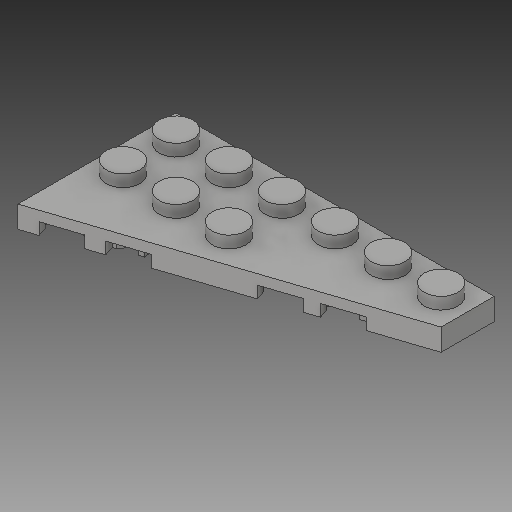
# Autodesk Inventor part: Grey triangle lego part
Saved by Autodesk Inventor 2017 (Build 210142000, 142)
## iProperties
Created: 2018-05-10
Part Number: Grey triangle lego part
Material: ABS Plastic
Document SubType Name: Modeling
Designer: 19000369
Density: 1.06 g/cm^3
Appearance: Light Gray
Mass: 1.84492 g
Surface Area: 27.5873 cm^2
Volume: 1.74049 cm^3
Author: 19000369
Autodesk Inventor part; units mm, degrees
ref_plane "YZ Plane" through (0, 0, 0) normal (1, 0, 0) x (0, 1, 0)
ref_plane "XZ Plane" through (0, 0, 0) normal (0, 1, 0) x (-1, 0, 0)
ref_plane "XY Plane" through (0, 0, 0) normal (0, 0, 1) x (1, 0, 0)
sketch "Sketch1" plane through (0, 0, 0) normal (0, 1, 0) x (-1, 0, 0)
  line L0 (0, 0) -> (0, -7.8486)
  line L1 (0, -7.8486) -> (47.0611, -7.8486)
  line L2 (47.0611, -7.8486) -> (47.0611, 15.5448)
  line L3 (47.0611, 15.5448) -> (0, 0)
  dimension "d0" = 7.8486
  dimension "d1" = 47.0611
  dimension "d2" = 23.3934
  constraints: 8 end point, 2 perpendicular, 1 vertical
  measures "d0" distance of L0.start L0.end
  measures "d1" distance of L0.end L1.end
  measures "d2" distance of L1.end L2.end
extrude "Extrusion1" add sketch "Sketch1" along normal blind 3.236
sketch "Sketch2" plane through (0, 3.236, 0) normal (0, 1, 0) x (1, 0, 0)
  circle A0 centre (-43.1394, 3.9268) radius 2.4867
  line L0 (-47.0611, 7.8486) -> (-47.0611, -15.5448) projected
  line L1 (0, 7.8486) -> (-47.0611, 7.8486) projected
  circle A1 centre (-43.1394, -3.9167) radius 2.4867
  circle A2 centre (-35.2958, 3.9268) radius 2.4867
  circle A3 centre (-35.2958, -3.9167) radius 2.4867
  circle A4 centre (-27.4523, 3.9268) radius 2.4867
  circle A5 centre (-27.4523, -3.9167) radius 2.4867
  circle A6 centre (-19.6088, 3.9268) radius 2.4867
  circle A7 centre (-19.6088, -3.9167) radius 2.4867
  circle A8 centre (-11.7653, 3.9268) radius 2.4867
  circle A9 centre (-11.7653, -3.9167) radius 2.4867
  circle A10 centre (-3.9218, 3.9268) radius 2.4867
  circle A11 centre (-3.9218, -3.9167) radius 2.4867
  dimension "d6" = 3.9218
  dimension "d7" = 3.9218
  dimension "d10" = 7.8435
  dimension "d13" = 7.8435
  constraints: 12 centre point, 1 horizontal, 1 vertical, 22 other
  measures "d6" distance from line of L0 A0.centre
  measures "d7" distance from line of L1 A0.centre
  measures "d10" distance of A0.centre A1.centre
  measures "d13" distance of A0.centre A2.centre
extrude "Extrusion2" add sketch "Sketch2" along normal blind 1.7577 contours A0 | A1 | A2 | A3 | A4 | A5 | A6 | A8 | A10
shell "Shell1" thickness 1.4732 removed faces 1 at (-31.3741, 0, 2.5654)
sketch "Sketch3" plane through (-45.5879, 1.7628, -6.3754) normal (0, -1, 0) x (1, 0, 0)
  circle A0 centre (5.8482, 6.3754) radius 2.4879
  circle A1 centre (13.8227, 6.3754) radius 2.4879
  circle A2 centre (21.5603, 6.3754) radius 2.4879
  circle A3 centre (29.3769, 6.3754) radius 2.4879
  circle A4 centre (37.9041, 6.3754) radius 2.4879
  circle A5 centre (5.8482, 15.0941) radius 2.4879
  line L0 (0, 19.8821) -> (44.1147, 5.3105) projected
  circle A6 centre (13.8227, 15.3163) radius 2.4879
  circle A7 centre (37.9041, 6.3754) radius 3.2245
  circle A8 centre (29.3769, 6.3754) radius 3.2245
  circle A9 centre (21.5603, 6.3754) radius 3.2245
  circle A10 centre (13.8227, 6.3754) radius 3.2245
  circle A11 centre (5.8482, 6.3754) radius 3.2245
  circle A12 centre (5.8482, 15.0941) radius 3.2245
  circle A13 centre (13.8227, 15.3163) radius 3.2245
  line L1 (0, 19.8821) -> (44.1147, 5.3105) projected
  line L2 (16.8845, 14.305) -> (16.1851, 14.536)
  line L3 (11.4603, 16.0966) -> (10.5982, 16.3814)
  line L4 (8.355, 17.1224) -> (5.0427, 18.2164)
  line L5 (41.1277, 6.2972) -> (40.3864, 6.542)
  line L6 (36.0094, 7.9878) -> (35.2681, 8.2327)
  point P0 (45.5879, 6.3754)
  dimension "d32" = 6.4491
  dimension "d19" = 4.9759
  dimension "d20" = 4.9759
  dimension "d21" = 4.9759
  dimension "d22" = 4.9759
  dimension "d23" = 4.9759
  dimension "d24" = 4.9759
  dimension "d25" = 4.9759
  dimension "d26" = 6.4491
  dimension "d27" = 6.4491
  dimension "d28" = 6.4491
  dimension "d29" = 6.4491
  dimension "d30" = 6.4491
  dimension "d31" = 6.4491
  constraints: 13 centre point, 10 end point, 8 point on circle, 7 coincident, 4 point on line, 11 other
  measures "d19" diameter of A0
  measures "d20" diameter of A1
  measures "d21" diameter of A2
  measures "d22" diameter of A3
  measures "d23" diameter of A4
  measures "d24" diameter of A5
  measures "d25" diameter of A6
  measures "d26" diameter of A7
  measures "d27" diameter of A8
  measures "d28" diameter of A9
  measures "d29" diameter of A10
  measures "d30" diameter of A11
  measures "d31" diameter of A12
sketch "Sketch4" plane through (-45.5879, 1.7628, -6.3754) normal (0, -1, 0) x (1, 0, 0)
  line L0 (0, 19.8821) -> (44.1147, 5.3105) projected
  arc A0 (35.2976, 8.2229) -> (41.086, 6.3109) centre (37.8811, 6.3263) ccw
  arc A1 (36.0857, 7.9626) -> (40.3651, 6.5491) centre (37.9224, 6.3384) ccw
  point P0 (45.5879, 6.3754)
  constraints: 4 point on circle, 4 point on line, 2 centre point
extrude "Extrusion4" add sketch "Sketch4" along normal blind 1.7628 contours L0 A1 A0
sketch "Sketch5" plane through (-45.5879, 1.7628, -6.3754) normal (0, -1, 0) x (1, 0, 0)
  line L0 (0, 19.8821) -> (35.2976, 8.2229) projected
  arc A0 (10.753, 16.3303) -> (16.8828, 14.3055) centre (13.8179, 15.3179) ccw
  arc A1 (11.4872, 16.0877) -> (16.1867, 14.5355) centre (13.8276, 15.2832) ccw
  arc A2 (5.0393, 18.2176) -> (8.3539, 17.1227) centre (5.8407, 15.0789) ccw
  circle A3 centre (5.8407, 15.0789) radius 2.4914
  point P0 (45.5879, 6.3754)
  constraints: 6 point on circle, 6 point on line, 4 centre point, 1 coincident
extrude "Extrusion5" add sketch "Sketch3" along normal blind 1.7628 contours A12 L0 | A8 | A9 | A10 | A11 picked at (6.7094, 17.5863)
extrude "Extrusion6" add sketch "Sketch5" along normal blind 1.7628 contours L0 A1 A0
sketch "Sketch6" plane through (0, 0, 0) normal (0, -1, 0) x (1, 0, 0)
  line L0 (-45.5879, 13.5067) -> (-40.5452, 11.841) projected
  line L1 (-45.1576, 13.3646) -> (-44.6956, 14.7634)
  line L2 (-47.0611, 15.5448) -> (0, 0) projected
  line L3 (-44.6956, 14.7634) -> (-39.5945, 13.0785)
  line L4 (-39.5945, 13.0785) -> (-40.0566, 11.6796)
  line L5 (-40.0566, 11.6796) -> (-45.1576, 13.3646)
  line L6 (-37.7514, 10.9182) -> (-37.2893, 12.3171)
  line L7 (-37.7514, 10.9182) -> (-32.6504, 9.2333)
  line L8 (-37.2329, 10.747) -> (-34.8349, 9.9549) projected
  line L9 (-32.6504, 9.2333) -> (-32.1883, 10.6322)
  line L10 (-32.1883, 10.6322) -> (-37.2893, 12.3171)
  line L11 (-9.5022, 1.5872) -> (-5.2228, 0.1737) projected
  line L12 (-8.7796, 1.3485) -> (-13.8806, 3.0334)
  line L13 (-13.8806, 3.0334) -> (-13.4186, 4.4323)
  line L14 (-13.4186, 4.4323) -> (-8.3175, 2.7474)
  line L15 (-8.7796, 1.3485) -> (-8.3175, 2.7474)
  line L16 (-15.3347, 5.0652) -> (-15.7967, 3.6663)
  line L17 (-15.7967, 3.6663) -> (-20.8978, 5.3513)
  line L18 (-28.7051, 7.9301) -> (-10.2903, 1.8475) projected
  line L19 (-20.8978, 5.3513) -> (-20.4357, 6.7501)
  line L20 (-15.3347, 5.0652) -> (-20.4357, 6.7501)
  dimension "d41" = 5.3721
  dimension "d42" = 5.3721
  dimension "d43" = 5.3721
  dimension "d44" = 5.3721
  constraints: 32 end point, 5 perpendicular, 4 point on line, 2 collinear, 1 parallel, 13 other
  measures "d41" distance of L1.end L3.end
  measures "d42" distance of L6.start L7.end
  measures "d43" distance of L12.start L12.end
  measures "d44" distance of L16.end L17.end
extrude "Extrusion7" cut sketch "Sketch6" against normal blind 1.7628 contours L1 L2 L4 L5 L0 | L2 L9 L7 L6 | L2 L16 L17 L19 | L2 L15 L11 L12 L13
body "Solid1"
